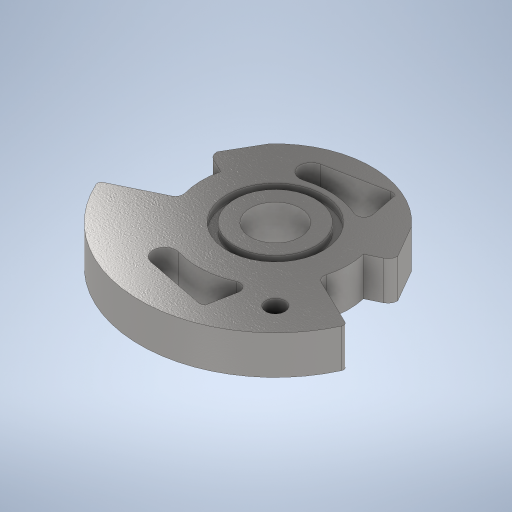
# Autodesk Inventor part: disc
Saved by Autodesk Inventor 2024 (Build 280153000, 153)
## iProperties
Created: 2024-02-09
Part Number: disc
Material: Stahl, galvanisiert
Document SubType Name: Modeling
Designer: ffogue
Density: 7.85 g/cm^3
Appearance: Galvanisiert
Author: ffogue
Autodesk Inventor part; units mm, degrees
ref_plane "XY Plane" through (0, 0, 0) normal (0, 0, 1) x (1, 0, 0)
sketch "Skizze1" plane through (0, 0, 0) normal (0, 0, 1) x (1, 0, 0)
  line L0 (0, 25) -> (0, -35) construction
  line L1 (-32.2, 0) -> (32.2, 0) construction
  circle A0 centre (0, 0) radius 19
  line L2 (-18.5027, 4.3188) -> (-24, 7)
  line L3 (-17.7846, -6.6863) -> (-32.2, -13.7171)
  line L4 (18.5027, 4.3188) -> (24, 7)
  line L5 (17.7846, -6.6863) -> (32.2, -13.7171)
  arc A1 (-32.2, -13.7171) -> (32.2, -13.7171) centre (0, 0) ccw
  arc A2 (24, 7) -> (-24, 7) centre (0, 0) ccw
  dimension "d3" = 38
  dimension "d4" = 26
  dimension "d5" = 52
  dimension "d6" = 26
  dimension "d7" = 52
  dimension "d8" = 48
  dimension "d9" = 64.4
  dimension "d10" = 60
  dimension "d11" = 25
  constraints: 12 end point, 10 point on circle, 3 centre point, 2 coincident, 2 horizontal alignment, 2 symmetric about line, 1 horizontal, 1 midpoint, 1 point on line, 1 vertical
  measures "d3" diameter of A0
  measures "d4" angle of L3 L1
  measures "d5" angle of L3 L2
  measures "d6" angle of L1 L4
  measures "d7" angle of L5 L4
  measures "d8" distance of L4.end L2.end
  measures "d9" distance of L5.end L3.end
  measures "d10" distance of L0.start L0.end
  measures "d11" radius of A2
extrude "Extrusion1" add sketch "Skizze1" along normal blind 10
fillet "Rundung1" radius 2.5 2 edges at (24, 7, 5) (-24, 7, 5)
sketch "Skizze2" plane through (0, 0, 10) normal (0, 0, 1) x (1, 0, 0)
  line L0 (0, 0) -> (24.7487, -24.7487) construction
  arc A0 (-32.2, -13.7171) -> (32.2, -13.7171) centre (0, 0) ccw projected
  line L1 (0, 0) -> (35, 0) construction
  point P0 (18.7383, -18.7383)
  dimension "d15" = 45
  dimension "d16" = 26.5
  constraints: 4 end point, 1 horizontal, 1 point on circle, 1 point on line
  measures "d15" angle of L1 L0
  measures "d16" distance of L0.start point (18.738, -18.738)
hole "Bohrung1" at (18.7383, -18.7383, 10) direction (0, 0, -1) diameter 5 end through all
fillet "Rundung2" radius 1 2 edges at (32.2, -13.7171, 5) (-32.2, -13.7171, 5)
fillet "Rundung3" radius 2 2 edges at (17.7846, -6.6863, 5) (-17.7846, -6.6863, 5)
sketch "Skizze3" plane through (0, 0, 10) normal (0, 0, 1) x (1, 0, 0)
  arc A0 (-23.2457, 9.1998) -> (-22.0171, 6.0329) centre (-20.9211, 8.2798) ccw projected
  line L0 (-23.4211, 8.2798) -> (-23.4211, 29.6928) construction
  line L1 (-23.4211, 8.2798) -> (-18.4816, 16.8354)
  line L2 (-23.4211, 8.2798) -> (-11.3111, 8.2798) construction
  arc A1 (23.2457, 9.1998) -> (-23.2457, 9.1998) centre (0, 0) ccw projected
  dimension "d27" = 30
  constraints: 6 end point, 2 point on circle, 1 horizontal, 1 tangent, 1 vertical
  measures "d27" angle of L1 L0
extrude "Extrusion2" cut sketch "Skizze3" against normal through all
ref_plane "Arbeitsebene1" through (0, 0, 0) normal (1, 0, 0) x (0, 1, 0)
mirror "Spiegeln1" about plane through (0, 0, 0) normal (1, 0, 0) of "Extrusion2"
sketch "Skizze4" plane through (0, 0, 10) normal (0, 0, 1) x (1, 0, 0)
  circle A0 centre (0, 0) radius 6.5
  dimension "d31" = 13
  constraints: 1 centre point, 1 coincident
  measures "d31" diameter of A0
extrude "Extrusion3" cut sketch "Skizze4" against normal blind 10
sketch "Skizze5" plane through (0, 0, 10) normal (0, 0, 1) x (1, 0, 0)
  circle A0 centre (0, 0) radius 10.5
  circle A1 centre (0, 0) radius 12.5
  dimension "d34" = 21
  dimension "d35" = 25
  constraints: 2 centre point, 2 coincident
  measures "d34" diameter of A0
  measures "d35" diameter of A1
extrude "Extrusion4" cut sketch "Skizze5" against normal blind 2
sketch "Skizze6" plane through (0, 0, 10) normal (0, 0, 1) x (1, 0, 0)
  arc A0 (-5.8207, -19.1299) -> (-7.2677, -24.9446) centre (-6.694, -22) ccw
  line L0 (-7.2677, -24.9446) -> (7.9346, -27.9063)
  arc A1 (7.9346, -27.9063) -> (9.4512, -27.5686) centre (8.306, -26) ccw
  line L1 (9.4512, -27.5686) -> (10.8468, -20.405)
  arc A2 (10.8468, -20.405) -> (8.1489, -18.2601) centre (8.9404, -20.0336) ccw
  arc A3 (-5.8207, -19.1299) -> (8.1489, -18.2601) centre (0, 0) ccw
  circle A4 centre (0, 0) radius 12.5 projected
  line L2 (0, 0) -> (0, -16.1046) construction
  dimension "d38" = 15
  dimension "d40" = 6
  dimension "d41" = 3
  dimension "d42" = 19.9959
  dimension "d43" = 22
  dimension "d44" = 26
  dimension "d45" = 20.0336
  constraints: 8 point on circle, 6 end point, 5 tangent, 4 centre point, 1 concentric, 1 equal radius, 1 perpendicular, 1 vertical, 3 other
  measures "d38" horizontal distance of A1.centre A0.centre
  measures "d40" distance of A2.centre A1.centre
  measures "d41" radius of A0
  measures "d42" radius of A3
  measures "d43" vertical distance of point (0, 0) A0.centre
  measures "d44" vertical distance of point (0, 0) A1.centre
  measures "d45" vertical distance of point (0, 0) A2.centre
extrude "Extrusion5" cut sketch "Skizze6" against normal up to surface (10 mm away) contours A3 A2 L1 A1 L0 A0
ref_plane "Arbeitsebene2" through (0, -3, 0) normal (0, 1, 0) x (-1, 0, 0)
mirror "Spiegeln2" about plane through (0, -3, 0) normal (0, 1, 0) of "Extrusion5"
